Autodesk Fusion 360 part; units mm, degrees
(part 2 of 2)
  line L272 (8.6409, -23.5874) -> (8.6409, -22.1855)
  spline S273 degree 3 poles (8.6409, -22.1855) (8.6409, -22.0708) (8.7341, -21.9781) (8.8484, -21.9781) knots 0 0 0 0 1 1 1 1
  line L273 (8.8484, -21.9781) -> (10.8857, -21.9781)
  spline S274 degree 3 poles (10.8857, -21.9781) (11, -21.9781) (11.0927, -22.0708) (11.0927, -22.1855) knots 0 0 0 0 1 1 1 1
  line L274 (11.0927, -22.1855) -> (11.0927, -23.5874)
  spline S275 degree 3 poles (11.0927, -23.5874) (11.0927, -23.7021) (11, -23.7949) (10.8857, -23.7949) knots 0 0 0 0 1 1 1 1
  line L275 (10.8857, -23.7949) -> (8.8484, -23.7949)
  spline S276 degree 3 poles (11.5401, -23.7949) (11.4261, -23.7949) (11.333, -23.7021) (11.333, -23.5874) knots 0 0 0 0 1 1 1 1
  line L276 (11.333, -23.5874) -> (11.333, -22.1855)
  spline S277 degree 3 poles (11.333, -22.1855) (11.333, -22.0708) (11.4261, -21.9781) (11.5401, -21.9781) knots 0 0 0 0 1 1 1 1
  line L277 (11.5401, -21.9781) -> (21.6031, -21.9781)
  spline S278 degree 3 poles (21.6031, -21.9781) (21.7177, -21.9781) (21.8105, -22.0708) (21.8105, -22.1855) knots 0 0 0 0 1 1 1 1
  line L278 (21.8105, -22.1855) -> (21.8105, -23.5874)
  spline S279 degree 3 poles (21.8105, -23.5874) (21.8105, -23.7021) (21.7177, -23.7949) (21.6031, -23.7949) knots 0 0 0 0 1 1 1 1
  line L279 (21.6031, -23.7949) -> (11.5401, -23.7949)
  spline S280 degree 3 poles (22.2553, -23.7949) (22.141, -23.7949) (22.0479, -23.7021) (22.0479, -23.5874) knots 0 0 0 0 1 1 1 1
  line L280 (22.0479, -23.5874) -> (22.0479, -22.1855)
  spline S281 degree 3 poles (22.0479, -22.1855) (22.0479, -22.0708) (22.141, -21.9781) (22.2553, -21.9781) knots 0 0 0 0 1 1 1 1
  line L281 (22.2553, -21.9781) -> (24.2693, -21.9781)
  spline S282 degree 3 poles (24.2693, -21.9781) (24.3836, -21.9781) (24.4768, -22.0708) (24.4768, -22.1855) knots 0 0 0 0 1 1 1 1
  line L282 (24.4768, -22.1855) -> (24.4768, -23.5874)
  spline S283 degree 3 poles (24.4768, -23.5874) (24.4768, -23.7021) (24.3836, -23.7949) (24.2693, -23.7949) knots 0 0 0 0 1 1 1 1
  line L283 (24.2693, -23.7949) -> (22.2553, -23.7949)
  spline S284 degree 3 poles (24.9216, -23.7949) (24.807, -23.7949) (24.7142, -23.7021) (24.7142, -23.5874) knots 0 0 0 0 1 1 1 1
  line L284 (24.7142, -23.5874) -> (24.7142, -22.1855)
  spline S285 degree 3 poles (24.7142, -22.1855) (24.7142, -22.0708) (24.807, -21.9781) (24.9216, -21.9781) knots 0 0 0 0 1 1 1 1
  line L285 (24.9216, -21.9781) -> (26.4118, -21.9781)
  spline S286 degree 3 poles (26.4118, -21.9781) (26.5261, -21.9781) (26.6192, -22.0708) (26.6192, -22.1855) knots 0 0 0 0 1 1 1 1
  line L286 (26.6192, -22.1855) -> (26.6192, -23.5874)
  spline S287 degree 3 poles (26.6192, -23.5874) (26.6192, -23.7021) (26.5261, -23.7949) (26.4118, -23.7949) knots 0 0 0 0 1 1 1 1
  line L287 (26.4118, -23.7949) -> (24.9216, -23.7949)
  spline S288 degree 3 poles (27.0641, -23.7949) (26.9498, -23.7949) (26.8566, -23.7021) (26.8566, -23.5874) knots 0 0 0 0 1 1 1 1
  line L288 (26.8566, -23.5874) -> (26.8566, -22.1855)
  spline S289 degree 3 poles (26.8566, -22.1855) (26.8566, -22.0708) (26.9498, -21.9781) (27.0641, -21.9781) knots 0 0 0 0 1 1 1 1
  line L289 (27.0641, -21.9781) -> (28.5542, -21.9781)
  spline S290 degree 3 poles (28.5542, -21.9781) (28.6688, -21.9781) (28.7616, -22.0708) (28.7616, -22.1855) knots 0 0 0 0 1 1 1 1
  line L290 (28.7616, -22.1855) -> (28.7616, -23.5874)
  spline S291 degree 3 poles (28.7616, -23.5874) (28.7616, -23.7021) (28.6688, -23.7949) (28.5542, -23.7949) knots 0 0 0 0 1 1 1 1
  line L291 (28.5542, -23.7949) -> (27.0641, -23.7949)
  spline S292 degree 3 poles (31.3485, -23.7949) (31.2342, -23.7949) (31.1415, -23.7021) (31.1415, -23.5874) knots 0 0 0 0 1 1 1 1
  line L292 (31.1415, -23.5874) -> (31.1415, -22.1855)
  spline S293 degree 3 poles (31.1415, -22.1855) (31.1415, -22.0708) (31.2342, -21.9781) (31.3485, -21.9781) knots 0 0 0 0 1 1 1 1
  line L293 (31.3485, -21.9781) -> (32.8394, -21.9781)
  spline S294 degree 3 poles (32.8394, -21.9781) (32.9533, -21.9781) (33.0465, -22.0708) (33.0465, -22.1855) knots 0 0 0 0 1 1 1 1
  line L294 (33.0465, -22.1855) -> (33.0465, -23.5874)
  spline S295 degree 3 poles (33.0465, -23.5874) (33.0465, -23.7021) (32.9533, -23.7949) (32.8394, -23.7949) knots 0 0 0 0 1 1 1 1
  line L295 (32.8394, -23.7949) -> (31.3485, -23.7949)
  spline S296 degree 3 poles (4.5635, -23.7949) (4.4492, -23.7949) (4.3561, -23.7021) (4.3561, -23.5874) knots 0 0 0 0 1 1 1 1
  line L296 (4.3561, -23.5874) -> (4.3561, -22.1855)
  spline S297 degree 3 poles (4.3561, -22.1855) (4.3561, -22.0708) (4.4492, -21.9781) (4.5635, -21.9781) knots 0 0 0 0 1 1 1 1
  line L297 (4.5635, -21.9781) -> (6.054, -21.9781)
  spline S298 degree 3 poles (6.054, -21.9781) (6.168, -21.9781) (6.2611, -22.0708) (6.2611, -22.1855) knots 0 0 0 0 1 1 1 1
  line L298 (6.2611, -22.1855) -> (6.2611, -23.5874)
  spline S299 degree 3 poles (6.2611, -23.5874) (6.2611, -23.7021) (6.168, -23.7949) (6.054, -23.7949) knots 0 0 0 0 1 1 1 1
  line L299 (6.054, -23.7949) -> (4.5635, -23.7949)
  spline S300 degree 3 poles (2.4208, -23.7949) (2.3068, -23.7949) (2.2137, -23.7021) (2.2137, -23.5874) knots 0 0 0 0 1 1 1 1
  line L300 (2.2137, -23.5874) -> (2.2137, -22.1855)
  spline S301 degree 3 poles (2.2137, -22.1855) (2.2137, -22.0708) (2.3068, -21.9781) (2.4208, -21.9781) knots 0 0 0 0 1 1 1 1
  line L301 (2.4208, -21.9781) -> (3.9112, -21.9781)
  spline S302 degree 3 poles (3.9112, -21.9781) (4.0259, -21.9781) (4.1187, -22.0708) (4.1187, -22.1855) knots 0 0 0 0 1 1 1 1
  line L302 (4.1187, -22.1855) -> (4.1187, -23.5874)
  spline S303 degree 3 poles (4.1187, -23.5874) (4.1187, -23.7021) (4.0259, -23.7949) (3.9112, -23.7949) knots 0 0 0 0 1 1 1 1
  line L303 (3.9112, -23.7949) -> (2.4208, -23.7949)
  spline S304 degree 3 poles (29.2061, -23.7949) (29.0922, -23.7949) (28.999, -23.7021) (28.999, -23.5874) knots 0 0 0 0 1 1 1 1
  line L304 (28.999, -23.5874) -> (28.999, -22.1855)
  spline S305 degree 3 poles (28.999, -22.1855) (28.999, -22.0708) (29.0922, -21.9781) (29.2061, -21.9781) knots 0 0 0 0 1 1 1 1
  line L305 (29.2061, -21.9781) -> (30.697, -21.9781)
  spline S306 degree 3 poles (30.697, -21.9781) (30.8109, -21.9781) (30.904, -22.0708) (30.904, -22.1855) knots 0 0 0 0 1 1 1 1
  line L306 (30.904, -22.1855) -> (30.904, -23.5874)
  spline S307 degree 3 poles (30.904, -23.5874) (30.904, -23.7021) (30.8109, -23.7949) (30.697, -23.7949) knots 0 0 0 0 1 1 1 1
  line L307 (30.697, -23.7949) -> (29.2061, -23.7949)
  line L308 (33.5901, -25.1103) -> (1.662, -25.1103)
  line L309 (1.662, -25.1103) -> (1.662, -10.492)
  line L310 (1.662, -10.492) -> (33.5901, -10.492)
  line L311 (33.5901, -10.492) -> (33.5901, -25.1103)
  line L312 (33.5901, -25.1103) -> (1.662, -10.492) construction
  line L313 (1.662, -25.1103) -> (33.5901, -10.492) construction
  point P0 (17.626, -17.8012)
  constraint horizontal L308
  constraint perpendicular L308 L309
  constraint parallel L308 L310
  constraint parallel L309 L311
  constraint coincident L312 P0
  constraint coincident L313 P0
  constraint midpoint L185 P0
extrude "Extrude2" add sketch "Key outlines" against normal blind 1 contours S0 L0 S1 L1 S2 L2 S3 L3 | S4 L4 S5 L5 S6 L6 S7 L7 | S8 L8 S9 L9 S10 L10 S11 L11 | S12 L12 S13 L13 S14 L14 S15 L15 | S16 L16 S17 L17 S18 L18 S19 L19 | S20 L20 S21 L21 S22 L22 S23 L23 | S24 L24 S25 L25 S26 L26 S27 L27 | S28 L28 S29 L29 S30 L30 S31 L31 | S32 L32 S33 L33 S34 L34 S35 L35 | S36 L36 S37 L37 S38 L38 S39 L39 | S40 L40 S41 L41 S42 L42 S43 L43 | S44 L44 S45 L45 S46 L46 S47 L47 | S48 L48 S49 L49 S50 L50 S51 L51 | S52 L52 S53 L53 S54 L54 S55 L55 | S56 L56 S57 L57 S58 L58 S59 L59 | S60 L60 S61 L61 S62 L62 S63 L63 | S64 L64 S65 L65 S66 L66 S67 L67 | S68 L68 S69 L69 S70 L70 S71 L71 | S72 L72 S73 L73 S74 L74 S75 L75 | S76 L76 S77 L77 S78 L78 S79 L79 | S80 L80 S81 L81 S82 L82 S83 L83 | S84 L84 S85 L85 S86 L86 S87 L87 | S88 L88 S89 L89 S90 L90 S91 L91 | S92 L92 S93 L93 S94 L94 S95 L95 | S96 L96 S97 L97 S98 L98 S99 L99 | S100 L100 S101 L101 S102 L102 S103 L103 | S104 L104 S105 L105 S106 L106 S107 L107 | S108 L108 S109 L109 S110 L110 S111 L111 | S112 L112 S113 L113 S114 L114 S115 L115 | S116 L116 S117 L117 S118 L118 S119 L119 | S120 L120 S121 L121 S122 L122 S123 L123 | S124 L124 S125 L125 S126 L126 S127 L127 | S128 L128 S129 L129 S130 L130 S131 L131 | S132 L132 S133 L133 S134 L134 S135 L135 | S136 L136 S137 L137 S138 L138 S139 L139 | S140 L140 S141 L141 S142 L142 S143 L143 | S144 L144 S145 L145 S146 L146 S147 L147 | S148 L148 S149 L149 S150 L150 S151 L151 | S152 L152 S153 L153 S154 L154 S155 L155 | S156 L156 S157 L157 S158 L158 S159 L159 | S160 L160 S161 L161 S162 L162 S163 L163 | S164 L164 S165 L165 S166 L166 S167 L167 | S168 L168 S169 L169 S170 L170 S171 L171 | S172 L172 S173 L173 S174 L174 S175 L175 | S176 L176 S177 L177 S178 L178 S179 L179 | S180 L180 S181 L181 S182 L182 S183 L183 | S184 L184 S185 L185 S186 L186 S187 L187 | S188 L188 S189 L189 S190 L190 S191 L191 | S192 L192 S193 L193 S194 L194 S195 L195 | S196 L196 S197 L197 S198 L198 S199 L199 | S200 L200 S201 L201 S202 L202 S203 L203 | S204 L204 S205 L205 S206 L206 S207 L207 | S208 L208 S209 L209 S210 L210 S211 L211 | S212 L212 S213 L213 S214 L214 S215 L215 | S216 L216 S217 L217 S218 L218 S219 L219 | S220 L220 S221 L221 S222 L222 S223 L223 | S224 L224 S225 L225 S226 L226 S227 L227 | S228 L228 S229 L229 S230 L230 S231 L231 | S232 L232 S233 L233 S234 L234 S235 L235 | S236 L236 S237 L237 S238 L238 S239 L239 | S240 L240 S241 L241 S242 L242 S243 L243 | S244 L244 S245 L245 S246 L246 S247 L247 | S248 L248 S249 L249 S250 L250 S251 L251 | S252 L252 S253 L253 S254 L254 S255 L255 | S256 L256 S257 L257 S258 L258 S259 L259 | S260 L260 S261 L261 S262 L262 S263 L263 | S264 L264 S265 L265 S266 L266 S267 L267 | S268 L268 S269 L269 S270 L270 S271 L271 | S272 L272 S273 L273 S274 L274 S275 L275 | S276 L276 S277 L277 S278 L278 S279 L279 | S280 L280 S281 L281 S282 L282 S283 L283 | S284 L284 S285 L285 S286 L286 S287 L287 | S288 L288 S289 L289 S290 L290 S291 L291 | S292 L292 S293 L293 S294 L294 S295 L295 | S296 L296 S297 L297 S298 L298 S299 L299 | S300 L300 S301 L301 S302 L302 S303 L303 | S304 L304 S305 L305 S306 L306 S307 L307 | L308 L309 L310 L311
extrude "Extrude3" cut sketch "Key outlines" against normal blind 0.5 contours S0 L0 S1 L1 S2 L2 S3 L3 | S4 L4 S5 L5 S6 L6 S7 L7 | S8 L8 S9 L9 S10 L10 S11 L11 | S12 L12 S13 L13 S14 L14 S15 L15 | S16 L16 S17 L17 S18 L18 S19 L19 | S20 L20 S21 L21 S22 L22 S23 L23 | S24 L24 S25 L25 S26 L26 S27 L27 | S28 L28 S29 L29 S30 L30 S31 L31 | S32 L32 S33 L33 S34 L34 S35 L35 | S36 L36 S37 L37 S38 L38 S39 L39 | S40 L40 S41 L41 S42 L42 S43 L43 | S44 L44 S45 L45 S46 L46 S47 L47 | S48 L48 S49 L49 S50 L50 S51 L51 | S52 L52 S53 L53 S54 L54 S55 L55 | S56 L56 S57 L57 S58 L58 S59 L59 | S60 L60 S61 L61 S62 L62 S63 L63 | S64 L64 S65 L65 S66 L66 S67 L67 | S68 L68 S69 L69 S70 L70 S71 L71 | S72 L72 S73 L73 S74 L74 S75 L75 | S76 L76 S77 L77 S78 L78 S79 L79 | S80 L80 S81 L81 S82 L82 S83 L83 | S84 L84 S85 L85 S86 L86 S87 L87 | S88 L88 S89 L89 S90 L90 S91 L91 | S92 L92 S93 L93 S94 L94 S95 L95 | S96 L96 S97 L97 S98 L98 S99 L99 | S100 L100 S101 L101 S102 L102 S103 L103 | S104 L104 S105 L105 S106 L106 S107 L107 | S108 L108 S109 L109 S110 L110 S111 L111 | S112 L112 S113 L113 S114 L114 S115 L115 | S116 L116 S117 L117 S118 L118 S119 L119 | S120 L120 S121 L121 S122 L122 S123 L123 | S124 L124 S125 L125 S126 L126 S127 L127 | S128 L128 S129 L129 S130 L130 S131 L131 | S132 L132 S133 L133 S134 L134 S135 L135 | S136 L136 S137 L137 S138 L138 S139 L139 | S140 L140 S141 L141 S142 L142 S143 L143 | S144 L144 S145 L145 S146 L146 S147 L147 | S148 L148 S149 L149 S150 L150 S151 L151 | S152 L152 S153 L153 S154 L154 S155 L155 | S156 L156 S157 L157 S158 L158 S159 L159 | S160 L160 S161 L161 S162 L162 S163 L163 | S164 L164 S165 L165 S166 L166 S167 L167 | S168 L168 S169 L169 S170 L170 S171 L171 | S172 L172 S173 L173 S174 L174 S175 L175 | S176 L176 S177 L177 S178 L178 S179 L179 | S180 L180 S181 L181 S182 L182 S183 L183 | S184 L184 S185 L185 S186 L186 S187 L187 | S188 L188 S189 L189 S190 L190 S191 L191 | S192 L192 S193 L193 S194 L194 S195 L195 | S196 L196 S197 L197 S198 L198 S199 L199 | S200 L200 S201 L201 S202 L202 S203 L203 | S204 L204 S205 L205 S206 L206 S207 L207 | S208 L208 S209 L209 S210 L210 S211 L211 | S212 L212 S213 L213 S214 L214 S215 L215 | S216 L216 S217 L217 S218 L218 S219 L219 | S220 L220 S221 L221 S222 L222 S223 L223 | S224 L224 S225 L225 S226 L226 S227 L227 | S228 L228 S229 L229 S230 L230 S231 L231 | S232 L232 S233 L233 S234 L234 S235 L235 | S236 L236 S237 L237 S238 L238 S239 L239 | S240 L240 S241 L241 S242 L242 S243 L243 | S244 L244 S245 L245 S246 L246 S247 L247 | S248 L248 S249 L249 S250 L250 S251 L251 | S252 L252 S253 L253 S254 L254 S255 L255 | S256 L256 S257 L257 S258 L258 S259 L259 | S260 L260 S261 L261 S262 L262 S263 L263 | S264 L264 S265 L265 S266 L266 S267 L267 | S268 L268 S269 L269 S270 L270 S271 L271 | S272 L272 S273 L273 S274 L274 S275 L275 | S276 L276 S277 L277 S278 L278 S279 L279 | S280 L280 S281 L281 S282 L282 S283 L283 | S284 L284 S285 L285 S286 L286 S287 L287 | S288 L288 S289 L289 S290 L290 S291 L291 | S292 L292 S293 L293 S294 L294 S295 L295 | S296 L296 S297 L297 S298 L298 S299 L299 | S300 L300 S301 L301 S302 L302 S303 L303 | S304 L304 S305 L305 S306 L306 S307 L307
fillet "Fillet1" radius 0.5 4 edges at (1.662, -25.1103, -0.5) (33.5901, -25.1103, -0.5) (1.662, -10.492, -0.5) (33.5901, -10.492, -0.5)
named bodies: "Keyboard wells"
